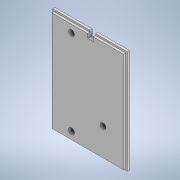
# Autodesk Inventor part: upper
Saved by Autodesk Inventor 2020 (Build 240168000, 168)
## iProperties
Created: 2020-04-03
Part Number: upper
Material: 일반
Document SubType Name: Modeling
Designer: orphe
Density: 1 g/cm^3
Appearance: 기본값
Author: orphe
Autodesk Inventor part; units mm, degrees
ref_plane "YZ Plane" through (0, 0, 0) normal (1, 0, 0) x (0, 1, 0)
ref_plane "XZ Plane" through (0, 0, 0) normal (0, 1, 0) x (-1, 0, 0)
ref_plane "XY Plane" through (0, 0, 0) normal (0, 0, 1) x (1, 0, 0)
sketch "스케치1" plane through (0, 0, 0) normal (0, 0, 1) x (1, 0, 0)
  line L0 (-32.5, 45) -> (32.5, 45)
  line L1 (32.5, 45) -> (32.5, -45)
  line L2 (32.5, -45) -> (-32.5, -45)
  line L3 (-32.5, -45) -> (-32.5, 45)
  line L4 (-32.5, 45) -> (32.5, -45) construction
  line L5 (32.5, 45) -> (-32.5, -45) construction
  point P0 (0, 0)
  dimension "d0" = 65
  dimension "d1" = 90
  constraints: 12 end point, 2 midpoint, 2 parallel, 1 horizontal, 1 perpendicular
  measures "d0" distance of L1.end L2.end
  measures "d1" distance of L0.end L1.end
extrude "돌출1" add sketch "스케치1" along normal blind 2
sketch "스케치3" plane through (0, 0, 2) normal (0, 0, 1) x (1, 0, 0)
  line L0 (-31, 43.5) -> (31, 43.5)
  line L1 (31, 43.5) -> (31, -43.5)
  line L2 (31, -43.5) -> (-31, -43.5)
  line L3 (-31, -43.5) -> (-31, 43.5)
  line L4 (-31, 43.5) -> (31, -43.5) construction
  line L5 (31, 43.5) -> (-31, -43.5) construction
  point P0 (0, 0)
  dimension "d8" = 62
  dimension "d9" = 87
  constraints: 12 end point, 2 midpoint, 2 parallel, 1 horizontal, 1 perpendicular
  measures "d8" distance of L1.end L2.end
  measures "d9" distance of L0.end L1.end
extrude "돌출3" add sketch "스케치3" along normal blind 2
sketch "스케치5" plane through (0, 0, 4) normal (0, 0, 1) x (1, 0, 0)
  line L0 (32.5, 45) -> (-32.5, 45) projected
  line L1 (0, 45) -> (5, 45)
  line L2 (5, 45) -> (5, 40)
  line L3 (5, 40) -> (0, 40)
  line L4 (0, 40) -> (0, 45)
  point P0 (0, 0)
  dimension "d14" = 5
  dimension "d15" = 5
  constraints: 8 end point, 2 parallel, 1 horizontal, 1 midpoint, 1 perpendicular
  measures "d14" distance of L2.end L3.end
  measures "d15" distance of L1.end L2.end
extrude "돌출4" cut sketch "스케치5" against normal blind 4
sketch "스케치6" plane through (0, 0, 4) normal (0, 0, 1) x (1, 0, 0)
  circle A0 centre (-14, 37) radius 2.5
  circle A1 centre (-14, -37) radius 2.5
  circle A2 centre (13.5, -19.5) radius 2.5
  point P0 (0, 0)
  dimension "d18" = 5
  dimension "d19" = 37
  dimension "d20" = 14
  dimension "d21" = 5
  dimension "d22" = 37
  dimension "d23" = 14
  dimension "d24" = 5
  dimension "d25" = 13.5
  dimension "d26" = 17.5
  constraints: 3 centre point
  measures "d18" diameter of A0
  measures "d19" vertical distance of point (0, 0) A0.centre
  measures "d20" horizontal distance of point (0, 0) A0.centre
  measures "d21" diameter of A1
  measures "d22" vertical distance of point (0, 0) A1.centre
  measures "d23" horizontal distance of point (0, 0) A1.centre
  measures "d24" diameter of A2
  measures "d25" horizontal distance of point (0, 0) A2.centre
  measures "d26" vertical distance of A1.centre A2.centre
extrude "돌출5" cut sketch "스케치6" against normal blind 4
